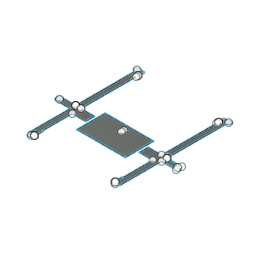
7F廊下用平面[少し幅大きく作ったから修正入れていこう] (Autodesk Fusion 360 design; units mm, degrees)
Autodesk Fusion 360 part; units mm, degrees
sketch "スケッチ1" plane through (0, 0, 0) normal (0, 0, 1) x (1, 0, 0)
  line L0 (10000, 0) -> (11000, 0)
  line L1 (11000, -4000) -> (0, -4000)
  line L2 (-63500, -29000.036) -> (-64000, -29000.036)
  line L3 (-63500, 42500) -> (-63500, 46500)
  line L4 (-54000, -6500.036) -> (-54000, -4000)
  line L5 (-64000, -34500.036) -> (-64000, -33000.036)
  line L6 (-34000, 2000) -> (-34000, 0)
  arc A0 (-79000, 0) -> (-79000, -4000) centre (-78000, -2000) ccw
  line L7 (-67000, -35000) -> (-68000, -35000)
  arc A1 (0, 43977.4822) -> (-1437.2284, 47000) centre (94.0203, 45875.1545) ccw
  line L8 (-64000, -6500.036) -> (-64000, -29000.036)
  line L9 (-64000, 42500) -> (-63500, 42500)
  line L10 (0, 41000) -> (0, 43977.4822)
  line L11 (-4500, -33000.036) -> (-4500, -29000.036)
  arc A2 (-67000, -35000) -> (-64000, -34500.036) centre (-65310.0198, -35889.9814) ccw
  arc A3 (-66562.7716, 47000) -> (-68000, 43977.4822) centre (-68094.0203, 45875.1545) ccw
  arc A4 (11000, -4000) -> (11000, 0) centre (10000, -2000) ccw
  line L12 (-79000, -4000) -> (-68000, -4000)
  line L13 (-68000, 41000) -> (-68000, 43977.4822)
  line L14 (11000, -4000) -> (0, -4000)
  line L15 (-1000, -35000) -> (0, -35000)
  line L16 (-64000, 46500) -> (-64000, 47000)
  line L17 (-64000, 0) -> (-64000, 42500)
  line L18 (-4000, 47000) -> (-1437.2284, 47000)
  line L19 (-78000, 0) -> (-79000, 0)
  line L20 (-68000, 0) -> (-78000, 0)
  line L21 (-4000, 0) -> (-4000, 42500)
  line L22 (-64000, -6500.036) -> (-54000, -6500.036)
  line L23 (-14000, -6500.036) -> (-14000, -4000)
  line L24 (-68000, 0) -> (-68000, 41000)
  line L25 (-63500, -33000.036) -> (-63500, -29000.036)
  line L26 (-4000, -6500.036) -> (-14000, -6500.036)
  line L27 (-4000, -33000.036) -> (-4500, -33000.036)
  line L28 (-4000, 42500) -> (-4500, 42500)
  line L29 (-68000, -4000) -> (-68000, -35000)
  line L30 (11000, 0) -> (0, 0)
  line L31 (-64000, -33000.036) -> (-63500, -33000.036)
  line L32 (0, -4000) -> (0, -35000)
  line L33 (-4500, 46500) -> (-4000, 46500)
  line L34 (-4000, 46500) -> (-4000, 47000)
  line L35 (0, 0) -> (10000, 0)
  line L36 (-64000, 47000) -> (-66562.7716, 47000)
  line L37 (-63500, 46500) -> (-64000, 46500)
  line L38 (-4000, -34500.036) -> (-4000, -33000.036)
  line L39 (-4000, -6500.036) -> (-4000, -29000.036)
  line L40 (-4500, -29000.036) -> (-4000, -29000.036)
  line L41 (-4500, 42500) -> (-4500, 46500)
  arc A5 (-4000, -34500.036) -> (-1000, -35000) centre (-2689.9802, -35889.9814) ccw
  line L42 (0, 0) -> (0, 41000)
  line L43 (-54000, -4000) -> (-54000, 0)
  line L44 (-54000, 0) -> (-64000, 0)
  line L45 (-4000, 0) -> (-14000, 0)
  line L46 (-14000, 0) -> (-14000, -4000)
  line L47 (-52000, 6000) -> (-16000, 6000)
  line L48 (-16000, 6000) -> (-16000, -15000)
  line L49 (-16000, -15000) -> (-52000, -15000)
  line L50 (-52000, -15000) -> (-52000, 6000)
  point P0 (-64000, 42500)
  point P1 (-64000, -6500.036)
  point P2 (-64000, 0)
  point P3 (-64000, -34500.036)
  point P4 (-68000, 0)
  point P5 (-64000, -35000)
  point P6 (-4000, 0)
  point P7 (-64000, 41000)
  point P8 (-4000, -35000)
  point P9 (-4000, 41000)
  point P10 (-4000, -6500.036)
  point P11 (-64000, 0)
  point P12 (-4000, 42500)
  point P13 (-4000, -34500.036)
  constraint parallel L4 L43
  constraint perpendicular L17 L44
  constraint perpendicular L21 L45
  constraint perpendicular L45 L46
  constraint horizontal L47
  constraint vertical L48
  constraint horizontal L49
  constraint vertical L50
extrude "押し出し1" add sketch "スケッチ1" along normal blind 10 contours L0 L1 A1 L10 L11 A4 L14 L15 L18 L21 L23 L26 L27 L28 L30 L32 L33 L34 L35 L38 L39 L40 L41 A5 L42 L45 L46 | L2 L3 L4 L5 A0 L7 L8 L9 A2 A3 L12 L13 L16 L17 L19 L20 L22 L24 L25 L29 L31 L36 L37 L43 L44 makes body 1 at (-10666.6667, -2166.6787, 10) makes body 2 at (-57333.3333, -4333.3573, 0)
extrude "押し出し2" add sketch "スケッチ1" against normal blind 10 separate body contours L47 L48 L49 L50 makes body 3
